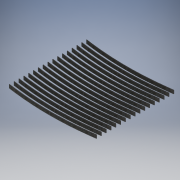
# Autodesk Inventor part: bent slat v2
Saved by Autodesk Inventor 2019 (Build 230136000, 136)
## iProperties
Created: 2018-08-04
Part Number: bent slat v2
Material: Steel
Document SubType Name: Modeling
Designer: torba
Density: 7.85 g/cm^3
Appearance: Plate
Author: torba
Autodesk Inventor part; units mm, degrees
ref_plane "YZ Plane" through (0, 0, 0) normal (1, 0, 0) x (0, 1, 0)
ref_plane "XZ Plane" through (0, 0, 0) normal (0, 1, 0) x (-1, 0, 0)
ref_plane "XY Plane" through (0, 0, 0) normal (0, 0, 1) x (1, 0, 0)
sketch "Sketch1" plane through (0, 0, 0) normal (0, 1, 0) x (-1, 0, 0)
  line L0 (577.9011, 30.8102) -> (574.7261, 30.8102)
  line L1 (571.5, 30.8102) -> (574.7261, 30.8102)
  line L2 (574.7571, 35.5727) -> (577.9321, 35.5727)
  line L3 (574.7571, 35.5727) -> (571.531, 35.5727)
  line L4 (-3.144, 0) -> (0.031, 0)
  line L5 (0, -4.7625) -> (3.175, -4.7625)
  line L6 (-104.775, -17.7825) -> (-104.775, -13.0238)
  line L7 (1254.125, -14.2136) -> (1254.125, -18.9803)
  line L8 (1146.175, -4.7498) -> (1149.35, -4.7498)
  line L9 (1149.381, 0.0127) -> (1152.556, 0.0127)
  arc A0 (1149.35, -4.7498) -> (0, -4.7625) centre (574.7261, -4629.7232) ccw
  line L10 (0.031, 0) -> (-104.775, -13.0238)
  line L11 (0, -4.7625) -> (-104.775, -17.7825)
  line L12 (1149.381, 0.0127) -> (1254.125, -14.2136)
  line L13 (1149.35, -4.7498) -> (1254.4891, -19.0298)
  line L14 (577.9321, 35.5727) -> (571.531, 35.5727)
  line L15 (577.9321, 35.5727) -> (577.9321, 35.5716)
  line L16 (571.531, 35.5727) -> (571.531, 35.5716)
  arc A1 (1149.381, 0.0127) -> (574.7571, 35.5727) centre (574.7571, -4624.9607) ccw
  arc A2 (571.531, 35.5716) -> (0.031, 0) centre (574.7571, -4624.9607) ccw
  point P0 (0, 0)
  dimension "d1" = 82.265
  dimension "d2" = 90
  dimension "d3" = 90
  dimension "d4" = 82.916
  dimension "d5" = 1358.9
  dimension "d6" = 4.7233
  dimension "d7" = 4.7625
  dimension "d8" = 35.56
  dimension "d9" = 30.7975
  dimension "d10" = 1254.125
  dimension "d11" = 149.9777
  dimension "d12" = 0.0127
  dimension "d13" = 0.3641
  dimension "d14" = 101.569
  dimension "d15" = 107.95
  dimension "d16" = 676.1929
  dimension "d17" = 676.2239
  dimension "d18" = 682.594
  dimension "d19" = 682.625
  dimension "d20" = 1250.95
  dimension "d21" = 1257.269
  constraints: 34 end point, 9 parallel, 8 point on circle, 4 tangent, 3 centre point, 1 horizontal, 1 perpendicular, 1 point on line, 1 vertical
  measures "d1" angle of L7 L13
  measures "d2" angle of L0 L7
  measures "d3" angle of L2 L7
  measures "d4" angle of L10 L7
  measures "d5" distance between parallel lines of L6 L7
  measures "d6" distance between parallel lines of L12 L13
  measures "d7" distance between parallel lines of L9 L8
  measures "d8" distance between parallel lines of L3 L9
  measures "d9" distance between parallel lines of L1 L9
  measures "d10" distance from line of point (0, 0) L7
  measures "d11" distance from line of point (0, 0) L13
  measures "d12" distance from line of point (0, 0) L9
  measures "d13" distance from line of L13.end L7
  measures "d14" distance from line of L9.end L7
  measures "d15" distance from line of L8.start L7
  measures "d16" distance from line of L2.end L7
  measures "d17" distance from line of L0.start L7
  measures "d18" distance from line of L3.end L7
  measures "d19" distance from line of L1.start L7
  measures "d20" distance from line of L5.end L7
  measures "d21" distance from line of L4.start L7
extrude "Extrusion1" add sketch "Sketch1" along normal blind 50.8
pattern_linear "Rectangular Pattern1" count 17 spacing 75.1078 along (0, 0, -1) of "Extrusion1"
body "Solid1"
